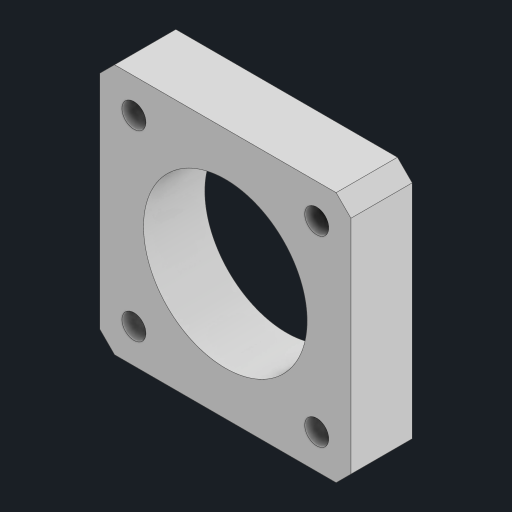
# Autodesk Inventor part: ArmEncoderSpacer
Saved by Autodesk Inventor 2023 (Build 270158000, 158)
## iProperties
Created: 2024-03-09
Part Number: ArmEncoderSpacer
Material: Generic
Document SubType Name: Modeling
Designer: valer
Density: 1 g/cm^3
Appearance: Default
Author: valer
Autodesk Inventor part; units mm, degrees
ref_plane "YZ Plane" through (0, 0, 0) normal (1, 0, 0) x (0, 1, 0)
ref_plane "XZ Plane" through (0, 0, 0) normal (0, 1, 0) x (-1, 0, 0)
ref_plane "XY Plane" through (0, 0, 0) normal (0, 0, 1) x (1, 0, 0)
sketch "Base" plane through (0, 0, 0) normal (0, 0, 1) x (1, 0, 0)
  circle A0 centre (-10.3744, 12.3744) radius 1.621 projected
  circle A1 centre (14.3744, 12.3744) radius 1.621 projected
  circle A2 centre (14.3743, -12.3743) radius 1.6234 projected
  circle A3 centre (-10.3742, -12.3743) radius 1.6233 projected
  line L0 (-19, -24.05) -> (-21, -22.05) construction
  line L1 (19, -24.05) -> (-19, -24.05) construction
  line L2 (21, -22.05) -> (19, -24.05) construction
  line L3 (21, 22.05) -> (21, -22.05) construction
  line L4 (19, 24.05) -> (21, 22.05) construction
  line L5 (19, 24.05) -> (-19, 24.05) construction
  line L6 (-21, 22.05) -> (-19, 24.05) construction
  line L7 (-21, -22.05) -> (-21, 22.05) construction
  circle A4 centre (2, 0) radius 11.075 projected
  circle A5 centre (14.3744, 12.3744) radius 1.621 projected
  circle A6 centre (-10.3744, 12.3744) radius 1.621 projected
  circle A7 centre (14.3744, -12.3744) radius 1.621 projected
  circle A8 centre (-10.3744, -12.3744) radius 1.621 projected
  line L8 (-12.7986, -9.12) -> (-8.0786, -9.12) construction
  line L9 (17, 17) -> (-13, 17) projected
  line L10 (-13, 17) -> (-15, 15) projected
  line L11 (-15, 15) -> (-15, -15) projected
  line L12 (-15, -15) -> (-13, -17) projected
  line L13 (-13, -17) -> (17, -17) projected
  line L14 (17, -17) -> (19, -15) projected
  line L15 (19, -15) -> (19, 15) projected
  line L16 (19, 15) -> (17, 17) projected
  point P0 (0, 0)
extrude "BaseFeature" add sketch "Base" against normal blind 8.3 contours L16 L15 L14 L13 L12 L11 L10 L9
body "Solid1"
